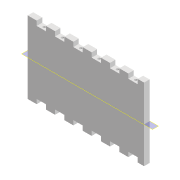
# Autodesk Inventor part: 00_Baseplate_Simmo_side6
Saved by Autodesk Inventor 2022 (Build 260153000, 153)
## iProperties
Created: 2022-05-05
Part Number: 00_Baseplate_Simmo_side6
Material: Generic
Document SubType Name: Modeling
Designer: wanghaoran
Density: 1 g/cm^3
Appearance: Default
Author: wanghaoran
Autodesk Inventor part; units mm, degrees
ref_plane "YZ Plane" through (0, 0, 0) normal (1, 0, 0) x (0, 1, 0)
ref_plane "XZ Plane" through (0, 0, 0) normal (0, 1, 0) x (-1, 0, 0)
ref_plane "XY Plane" through (0, 0, 0) normal (0, 0, 1) x (1, 0, 0)
sketch "Sketch1" plane through (0, 0, 0) normal (0, 0, 1) x (1, 0, 0)
  line L0 (0, -129) -> (0, 146.2673) projected
  line L1 (-130, -1) -> (-130, 5) projected
  line L2 (-10, 5) -> (0, 5) projected
  line L3 (0, -74) -> (-450, -74) projected
  line L4 (-130, 5) -> (-120, 5) projected
  line L5 (0, -74) -> (-129.8, -74) projected
  line L6 (-129.8, -68) -> (-129.8, -74) projected
  line L7 (0, 5) -> (-129.9001, 5)
  line L8 (-129.9001, 5) -> (-129.9001, -74)
  line L9 (-129.9001, -74) -> (0, -74)
  line L10 (0, -74) -> (0, 5)
  line L11 (-155.5538, 0) -> (-155.5538, 5) projected
  line L12 (-170.1, 0) -> (-170.1, 5) projected
  point P0 (0, 0)
  point P1 (-129.9001, -74)
  point P2 (-120, 5)
  point P3 (-130, 0)
  point P4 (-129.9001, 5)
  point P5 (-129.9001, 5)
  constraints: 8 end point, 2 parallel, 1 horizontal, 1 perpendicular
extrude "Extrusion1" add sketch "Sketch1" along normal blind 6
ref_plane "Work Plane2" through (-20.1, 0, 6) normal (0, 1, 0) x (1, 0, 0)
sketch "Sketch3" plane through (-20.1, 0, 6) normal (0, 1, 0) x (1, 0, 0)
  circle A0 centre (5.1, 3) radius 1.5 projected
  point P0 (20.1, 6)
hole "Hole1" at (-15, 0, 3) direction (0, -1, 0) diameter 2.8 depth 20
ref_plane "Work Plane1" through (-129.9001, -34.5, 0) normal (0, -1, 0) x (1, 0, 0)
sketch "Skizze4" plane through (0, 0, 6) normal (0, 0, 1) x (1, 0, 0)
  line L0 (-2.3877, -54.9) -> (-2.3877, -60) projected
  line L1 (16.4895, -81.7963) -> (-2.8877, -81.7963)
  line L2 (-2.8877, -81.7963) -> (-2.8877, 13.3495)
  line L3 (-2.8877, 13.3495) -> (16.4895, 13.3495)
  line L4 (16.4895, 13.3495) -> (16.4895, -81.7963)
  point P0 (0, 0)
  dimension "d23" = 0.5
  constraints: 8 end point, 2 parallel, 1 horizontal, 1 perpendicular
  measures "d23" distance between parallel lines of L0 L2
extrude "Extrusion3" cut sketch "Skizze4" against normal blind 10
sketch "Sketch6" plane through (0, 0, 6) normal (0, 0, 1) x (1, 0, 0)
  line L0 (-100, 5) -> (-100, -1) projected
  line L1 (-100, -1) -> (-90, -1) projected
  line L2 (-90, -1) -> (-90, 5) projected
  line L3 (-2.8877, 5) -> (-129.9001, 5) projected
  point P0 (0, 0)
  point P1 (-100, 5)
  point P2 (-90, 5)
extrude "Extrusion5" cut sketch "Sketch6" against normal through all
pattern_linear "Rectangular Pattern3" count 3 spacing 20 along (1, 0, 0) of "Extrusion5"
body "Solid1"
